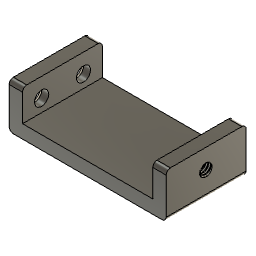
Full Assembled Design (Autodesk Fusion 360 archive; units mm, degrees)
design "C Bracket Updated"
Autodesk Fusion 360 part; units mm, degrees
sketch "Sketch1" plane through (0, 0, 0) normal (0, 0, 1) x (1, 0, 0)
  line L0 (31, 19) -> (-31, 19)
  line L1 (-31, 19) -> (-31, -19)
  line L2 (-31, -19) -> (31, -19)
  line L3 (31, -19) -> (31, 19)
  line L4 (31, 19) -> (-31, -19) construction
  line L5 (-31, 19) -> (31, -19) construction
  line L6 (31, 19) -> (37.35, 19)
  line L7 (37.35, 19) -> (37.35, -19)
  line L8 (37.35, -19) -> (31, -19)
  line L9 (31, -19) -> (31, 19)
  line L10 (-31, -19) -> (-37.35, -19)
  line L11 (-37.35, -19) -> (-37.35, 19)
  line L12 (-37.35, 19) -> (-31, 19)
  line L13 (-31, 19) -> (-31, -19)
  dimension "d1" = 38
  dimension "d2" = 62
  dimension "d3" = 6.35
  dimension "d4" = 38
  dimension "d5" = 6.35
  dimension "d6" = 38
  constraint horizontal L0
  constraint perpendicular L0 L1
  constraint parallel L0 L2
  constraint parallel L1 L3
  constraint coincident L4 origin
  constraint coincident L5 origin
  constraint horizontal L6
  constraint vertical L7
  constraint horizontal L8
  constraint vertical L9
  constraint horizontal L10
  constraint vertical L11
  constraint horizontal L12
  constraint vertical L13
  measures "d1" distance of L0.end L1.end
  measures "d2" distance of L1.end L2.end
  measures "d3" distance of L0.start L6.end
  measures "d4" distance of L0.start L2.end
  measures "d5" distance of L1.end L10.end
  measures "d6" distance of L1.end L0.end
extrude "Extrude1" add sketch "Sketch1" against normal blind 6.35
extrude "Extrude2" add sketch "Sketch1" along normal blind 15 contours L3 L6 L7 L8 L9 | L1 L10 L11 L12 L13
fillet "Fillet1" radius 2 2 edges at (37.35, 0, -6.35) (-37.35, 0, -6.35)
fillet "Fillet2" radius 2 4 edges at (-34.175, 19, 15) (-34.175, -19, 15) (34.175, -19, 15) (34.175, 19, 15)
sketch "Sketch2" plane through (37.35, 0, 0) normal (1, 0, 0) x (0, 1, 0)
  arc A0 (19, 13) -> (17, 15) centre (17, 13) ccw
  line L0 (17, 15) -> (-17, 15)
  arc A1 (-17, 15) -> (-19, 13) centre (-17, 13) ccw
  line L1 (-19, 13) -> (-19, -4.35)
  line L2 (-19, -4.35) -> (19, -4.35)
  line L3 (19, -4.35) -> (19, 13)
  circle A2 centre (0, 6) radius 3.3782
  dimension "d15" = 6.7564
  dimension "d16" = 9
  measures "d15" diameter of A2
  measures "d16" distance of L0 A2.centre
extrude "Extrude3" cut sketch "Sketch2" against normal blind 22 contours A2
sketch "Sketch3" plane through (-37.35, 0, 0) normal (-1, 0, 0) x (0, -1, 0)
  arc A0 (19, 13) -> (17, 15) centre (17, 13) ccw
  line L0 (17, 15) -> (-17, 15)
  arc A1 (-17, 15) -> (-19, 13) centre (-17, 13) ccw
  line L1 (-19, 13) -> (-19, -4.35)
  line L2 (-19, -4.35) -> (19, -4.35)
  line L3 (19, -4.35) -> (19, 13)
  circle A2 centre (-10, 6) radius 3.38
  line L4 (-0.0396, -11.2502) -> (-0.0396, 20.5797) construction
  circle A3 centre (9.9207, 6) radius 3.38
  dimension "d19" = 6.76
  dimension "d20" = 9
  dimension "d21" = 9
  constraint perpendicular L0 L4
  constraint symmetric A2 L4 A3
  measures "d19" diameter of A2
  measures "d20" distance of L1 A2.centre
  measures "d21" distance of L0 A2.centre
extrude "Extrude4" cut sketch "Sketch3" against normal blind 12 contours A2 | A3
chamfer "Chamfer1" distance 3.03 distance2 3.03 2 edges at (-37.35, 13.1513, 7.2223) (-37.35, -6.7695, 7.2223) measured on face at (-37.35, -2.8953, -1.9488) measured on face at (-37.35, -2.8953, -1.9488)
thread "Thread1" "ANSI Unified Screw Threads 0.25 1/4-20 UNC 3B" major diameter 6.35 minor diameter 5.1156 pitch 1.27 angle 60 modelled right hand crest width 0.3725 on face at (33.1167, 3.3614, 5.6636) crest through (37.0325, 2.5578, 6)

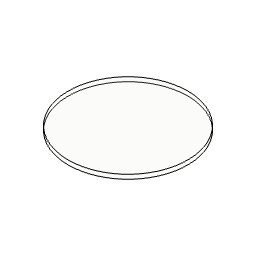
design "CBA Top Cover"
Autodesk Fusion 360 part; units mm, degrees
sketch "Sketch1" plane through (0, 0, 0) normal (0, 0, 1) x (1, 0, 0)
  circle A0 centre (0, 0) radius 41.5
  dimension "d1" = 83
  constraint coincident A0.centre origin
  measures "d1" diameter of A0
extrude "Extrude1" add sketch "Sketch1" along normal blind 3
named bodies: "CBA Top Cover"

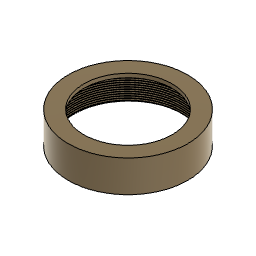
design "CBA Rim"
Autodesk Fusion 360 part; units mm, degrees
sketch "Sketch1" plane through (0, 0, 0) normal (0, 0, 1) x (1, 0, 0)
  circle A0 centre (0, 0) radius 46
  dimension "d1" = 92
  constraint coincident A0.centre origin
  measures "d1" diameter of A0
extrude "Extrude1" add sketch "Sketch1" along normal blind 21.5 makes body 1
sketch "Sketch3" plane through (0, 0, 21.5) normal (0, 0, 1) x (-1, 0, 0)
  circle A0 centre (0, 0) radius 46
  circle A1 centre (0, 0) radius 34
  dimension "d9" = 12
  constraint coincident A0.centre A1.centre
  measures "d9" distance of A0 A1
extrude "Extrude3" add sketch "Sketch3" along normal blind 3 separate body makes body 2
sketch "Sketch4" plane through (0, 0, 0) normal (0, 0, -1) x (1, 0, 0)
  circle A0 centre (0, 0) radius 46
  circle A1 centre (0, 0) radius 34
  dimension "d12" = 68
  constraint coincident A0.centre A1.centre
  measures "d12" diameter of A1
extrude "Extrude4" cut sketch "Sketch4" against normal blind 21.5 contours A1 bodies 1
thread "Thread2" "ISO Metric profile 85.0 M85x1.5 6H" major diameter 85.2143 minor diameter 83.5262 pitch 1.5 angle 60 modelled right hand crest width 0.4004 on face at (33.9577, 1.6948, 14.3333) crest through (41.7631, 0, 0.375) on bodies 1
combine "Combine1" operation add target body 2 tool bodies 1
named bodies: "CBA Rim"

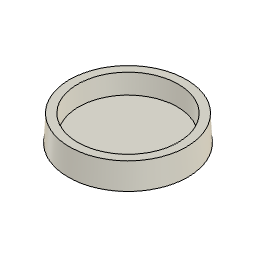
design "PDMS Substrate"
Autodesk Fusion 360 part; units mm, degrees
sketch "Sketch1" plane through (0, 0, 0) normal (0, 0, 1) x (1, 0, 0)
  circle A0 centre (0, 0) radius 29
  dimension "d1" = 58
  constraint coincident A0.centre origin
  measures "d1" diameter of A0
extrude "Extrude1" add sketch "Sketch1" along normal blind 12.7
sketch "Sketch2" plane through (0, 0, 12.7) normal (0, 0, 1) x (-1, 0, 0)
  circle A0 centre (0, 0) radius 29
  circle A1 centre (0, 0) radius 25
  dimension "d4" = 50
  constraint concentric A0 A1
  measures "d4" diameter of A1
extrude "Extrude2" cut sketch "Sketch2" against normal blind 9.5 contours A1
draft "Draft1" angle 3 neutral plane through (0, 0, 12.7) pull (0, 0, 1) 1 faces at (-28.8559, 2.8875, 4.2333)
draft "Draft2" angle 3 neutral plane through (0, 0, 12.7) pull (0, 0, 1) 1 faces at (-24.8758, 2.4892, 6.3667)
named bodies: "PDMS Substrate"

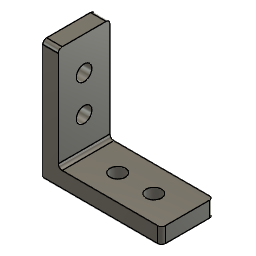
design "90deg_bracket"
Autodesk Fusion 360 part; units mm, degrees
sketch "Sketch1" plane through (0, 0, 0) normal (0, 0, 1) x (1, 0, 0)
  line L0 (0, 0) -> (-6, 0)
  line L1 (-6, 0) -> (-6, 46)
  line L2 (-6, 46) -> (0, 46)
  line L3 (0, 46) -> (0, 0)
  line L4 (0, 0) -> (40, 0)
  line L5 (40, 0) -> (40, 6)
  line L6 (40, 6) -> (0, 6)
  line L7 (0, 6) -> (0, 0)
  dimension "d1" = 6
  dimension "d2" = 46
  dimension "d3" = 40
  dimension "d4" = 6
  constraint horizontal L0
  constraint vertical L1
  constraint horizontal L2
  constraint vertical L3
  constraint coincident L0.start L3.end
  constraint horizontal L4
  constraint vertical L5
  constraint horizontal L6
  constraint vertical L7
  measures "d1" distance of L0.start L0.end
  measures "d2" distance of L0.start L2.end
  measures "d3" distance of L0.start L4.end
  measures "d4" distance of L0.start L6.end
extrude "Extrude1" add sketch "Sketch1" along normal blind 20
fillet "Fillet1" radius 1.5 4 edges at (40, 3, 20) (-3, 46, 20) (-3, 46, 0) (40, 3, 0)
sketch "Sketch2" plane through (0, 6, 0) normal (0, 1, 0) x (-1, 0, 0)
  arc A0 (-40, 1.5) -> (-38.5, 0) centre (-38.5, 1.5) ccw
  line L0 (-38.5, 0) -> (0, 0)
  line L1 (0, 0) -> (0, 20)
  line L2 (0, 20) -> (-38.5, 20)
  arc A1 (-38.5, 20) -> (-40, 18.5) centre (-38.5, 18.5) ccw
  line L3 (-40, 18.5) -> (-40, 1.5)
  circle A2 centre (-13, 10) radius 3
  circle A3 centre (-27, 10) radius 3
  point P0 (-19.25, 10)
  dimension "d11" = 6
  dimension "d12" = 6
  measures "d11" diameter of A2
  measures "d12" diameter of A3
sketch "Sketch3" plane through (0, 0, 0) normal (1, 0, 0) x (0, 0, -1)
  arc A0 (0, 44.5) -> (-1.5, 46) centre (-1.5, 44.5) ccw
  line L0 (-1.5, 46) -> (-18.5, 46)
  arc A1 (-18.5, 46) -> (-20, 44.5) centre (-18.5, 44.5) ccw
  line L1 (-20, 44.5) -> (-20, 6)
  line L2 (-20, 6) -> (0, 6)
  line L3 (0, 6) -> (0, 44.5)
  circle A2 centre (-10, 33) radius 3
  circle A3 centre (-10, 19) radius 3
  dimension "d15" = 6
  dimension "d16" = 6
  measures "d15" diameter of A2
  measures "d16" diameter of A3
extrude "Extrude2" cut sketch "Sketch2" against normal blind 7 contours A2 | A3
extrude "Extrude3" cut sketch "Sketch3" against normal blind 7 contours A2 | A3
fillet "Fillet2" radius 1.5 1 edges at (0, 6, 10)

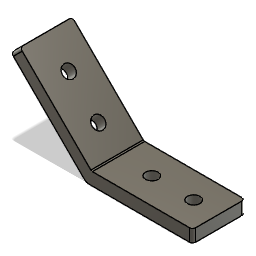
design "45deg_bracket"
Autodesk Fusion 360 part; units mm, degrees
sketch "Sketch1" plane through (0, 0, 0) normal (0, 0, 1) x (1, 0, 0)
  line L0 (0, 0) -> (-50.8, 0)
  line L1 (-48.3147, 6) -> (0, 6)
  line L2 (0, 6) -> (0, 0)
  line L3 (-50.8, 0) -> (-86.721, 35.921)
  line L4 (-48.3147, 6) -> (-82.4728, 40.158)
  line L5 (-82.4728, 40.158) -> (-86.721, 35.921)
  dimension "d1" = 50.8
  dimension "d2" = 6
  dimension "d3" = 135
  dimension "d4" = 135
  dimension "d5" = 6
  dimension "d6" = 50.8
  constraint horizontal L0
  constraint horizontal L1
  constraint vertical L2
  constraint coincident L0.start L2.end
  measures "d1" distance of L0.start L0.end
  measures "d2" distance of L0.start L1.end
  measures "d3" angle of L0 L3
  measures "d4" angle of L1 L4
  measures "d5" distance of L3.end L4.end
  measures "d6" distance of L0.end L3.end
extrude "Extrude1" add sketch "Sketch1" against normal blind 25
fillet "Fillet1" radius 1 1 edges at (-48.3147, 6, -12.5)
fillet "Fillet1" radius 3 1 edges at (-50.8, 0, -12.5)
sketch "Sketch2" plane through (-21.1574, -21.1574, 0) normal (0.707107, 0.707107, 0) x (0, 0, -1)
  line L0 (0, 38.8205) -> (25, 38.8205)
  line L1 (25, 38.8205) -> (25, 86.7131)
  line L2 (25, 86.7131) -> (0, 86.7131)
  line L3 (0, 86.7131) -> (0, 38.8205)
  line L4 (0, 62.7668) -> (25, 62.7668)
  line L5 (25, 62.7668) -> (25, 86.7131)
  line L6 (0, 38.8205) -> (0, 62.7668)
  line L7 (0, 50.7937) -> (25, 50.7937)
  circle A0 centre (12.5, 51.4569) radius 3
  circle A1 centre (12.5, 71.4569) radius 3
  line L8 (12.5, 86.7131) -> (12.5, 38.8205)
  line L9 (12.5, 71.4569) -> (12.5, 51.4569)
  dimension "d14" = 6
  dimension "d15" = 6
  dimension "d24" = 20
  constraint midpoint L3 L4.start
  constraint midpoint L1 L4.end
  constraint coincident L1.end L2.start
  constraint coincident L0.start L3.end
  constraint midpoint L6 L7.start
  constraint coincident L1 L7.end
  constraint perpendicular L1 L7
  constraint midpoint L2 L8.start
  constraint midpoint L0 L8.end
  constraint coincident A1.centre L8
  constraint coincident A1.centre L9.start
  constraint parallel L8 L9
  constraint coincident A0.centre L9.end
  measures "d14" diameter of A0
  measures "d15" diameter of A1
  measures "d24" distance of A1.centre A0.centre
sketch "Sketch3" plane through (0, 6, 0) normal (0, 1, 0) x (-1, 0, 0)
  line L0 (47.9005, -25) -> (47.9005, 0)
  line L1 (47.9005, 0) -> (0, 0)
  line L2 (0, 0) -> (0, -25)
  line L3 (0, -25) -> (47.9005, -25)
  line L4 (23.9503, 0) -> (23.9503, -25)
  line L5 (23.9503, 0) -> (47.9005, 0)
  line L6 (23.9503, 0) -> (0, 0)
  line L7 (11.9751, 0) -> (11.9751, -25)
  circle A0 centre (31.9751, -12.5) radius 3
  circle A1 centre (11.9751, -12.5) radius 3
  line L8 (0, -12.5) -> (47.9005, -12.5)
  line L9 (31.9751, -12.5) -> (11.9751, -12.5)
  dimension "d16" = 6
  dimension "d17" = 6
  dimension "d25" = 20
  constraint midpoint L1 L4.start
  constraint perpendicular L1 L4
  constraint coincident L0.end L1.start
  constraint coincident L1.end L2.start
  constraint midpoint L6 L7.start
  constraint coincident L3 L7.end
  constraint perpendicular L3 L7
  constraint midpoint L2 L8.start
  constraint midpoint L0 L8.end
  constraint midpoint L7 A1.centre
  constraint coincident A0.centre L9.start
  constraint coincident A1.centre L9.end
  constraint perpendicular L7 L9
  measures "d16" diameter of A0
  measures "d17" diameter of A1
  measures "d25" distance of A0.centre A1.centre
extrude "Extrude2" cut sketch "Sketch3" against normal blind 6 contours A0 L8 L9 | A0 L8 L9 | L7 A1 L8 | L7 A1 L8 L9 | L7 A1 L8 L9 | L7 A1 L8
extrude "Extrude3" cut sketch "Sketch2" against normal blind 6 contours L7 A0 L8 | L7 A0 L8 | L7 A0 L8 L9 | L7 A0 L8 L9 | A1 L8 L9 | A1 L8 L9
fillet "Fillet2" radius 1.5 4 edges at (-84.5969, 38.0395, -25) (-84.5969, 38.0395, 0) (0, 3, 0) (0, 3, -25)
